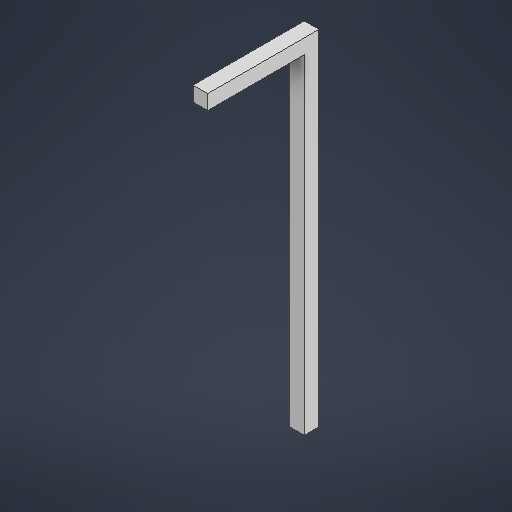
# Autodesk Inventor part: switch-wire
Saved by Autodesk Inventor 2025.2 (Build 292293000, 293)
## iProperties
Created: 2025-12-13
Part Number: switch-wire
Material: Generic
Document SubType Name: Modeling
Designer: sam
Density: 1 g/cm^3
Appearance: Default
Author: sam
Autodesk Inventor part; units mm, degrees
ref_plane "YZ Plane" through (0, 0, 0) normal (1, 0, 0) x (0, 1, 0)
ref_plane "XZ Plane" through (0, 0, 0) normal (0, 1, 0) x (-1, 0, 0)
ref_plane "XY Plane" through (0, 0, 0) normal (0, 0, 1) x (1, 0, 0)
sketch "Sketch1" plane through (0, 0, 0) normal (0, 1, 0) x (-1, 0, 0)
  line L0 (0.25, 0.25) -> (-0.25, 0.25)
  line L1 (-0.25, 0.25) -> (-0.25, -0.25)
  line L2 (-0.25, -0.25) -> (0.25, -0.25)
  line L3 (0.25, -0.25) -> (0.25, 0.25)
  line L4 (0.25, 0.25) -> (-0.25, -0.25) construction
  line L5 (-0.25, 0.25) -> (0.25, -0.25) construction
  point P0 (0, 0)
  dimension "d0" = 0.5
  dimension "d1" = 0.5
  constraints: 12 end point, 2 midpoint, 2 parallel, 1 horizontal, 1 perpendicular
  measures "d0" distance of L2.end L1.end
  measures "d1" distance of L1.end L0.end
extrude "Extrusion1" add sketch "Sketch1" along normal blind 11.75
sketch "Sketch2" plane through (-0.25, 0, 0.25) normal (0, 0, 1) x (1, 0, 0)
  line L0 (0, 0) -> (0.5, 0) projected
  line L1 (0.5, 0) -> (0.5, 11.75) projected
  line L2 (0, 11.75) -> (0.5, 11.75) projected
  line L3 (0, 0) -> (0, 11.75) projected
  line L4 (0, 11.75) -> (0.5, 11.75)
  line L5 (0.5, 11.75) -> (0.5, 11.25)
  line L6 (0.5, 11.25) -> (0, 11.25)
  line L7 (0, 11.25) -> (0, 11.75)
  point P0 (0.25, 0)
  point P1 (0, 11.25)
  dimension "d10" = 0.5
  constraints: 8 end point, 2 parallel, 1 horizontal, 1 perpendicular, 1 point on line
  measures "d10" distance of L4.end L5.end
extrude "Extrusion2" add sketch "Sketch2" along normal blind 3.3 contours L3 L2 L1 L6
body "Solid1"
